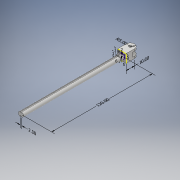
# Autodesk Inventor part: Tige
Saved by Autodesk Inventor 2018 (Build 220112000, 112)
## iProperties
Created: 2018-03-30
Part Number: Tige
Material: Générique
Document SubType Name: Modeling
Designer: Guadalix
Density: 1 g/cm^3
Appearance: Par défaut
Author: Guadalix
Autodesk Inventor part; units mm, degrees
ref_plane "YZ Plane" through (0, 0, 0) normal (1, 0, 0) x (0, 1, 0)
ref_plane "XZ Plane" through (0, 0, 0) normal (0, 1, 0) x (-1, 0, 0)
ref_plane "XY Plane" through (0, 0, 0) normal (0, 0, 1) x (1, 0, 0)
sketch "Esquisse1" plane through (0, 0, 0) normal (0, 0, 1) x (1, 0, 0)
  line L0 (-5, -5) -> (5, -5)
  line L1 (5, -5) -> (5, 5)
  line L2 (5, 5) -> (-5, 5)
  line L3 (-5, 5) -> (-5, -5)
  line L4 (-5, -5) -> (5, 5) construction
  line L5 (5, -5) -> (-5, 5) construction
  arc A0 (5, 5) -> (-5, 5) centre (0, 5) ccw
  point P0 (0, 0)
  dimension "d0" = 10
  dimension "d1" = 10
  constraints: 12 end point, 2 midpoint, 2 parallel, 2 point on circle, 1 centre point, 1 horizontal, 1 perpendicular, 1 tangent
  measures "d0" distance of L1.end L2.end
  measures "d1" distance of L0.end L1.end
extrude "Extrusion1" add sketch "Esquisse1" along normal blind 10
hole "Perçage1" at (0, 5, 10) direction (0, 0, -1) diameter 3 end through all
sketch "Esquisse3" plane through (0, 0, 0) normal (1, 0, 0) x (0, 1, 0)
  line L0 (15, 0) -> (15, 10)
  line L1 (3, 0) -> (3, 10)
  line L2 (15, 2.5) -> (3, 2.5)
  line L3 (3, 2.5) -> (3, 7.5)
  line L4 (3, 7.5) -> (15, 7.5)
  line L5 (15, 7.5) -> (15, 2.5)
  line L6 (15, 10) -> (3, 10)
  line L7 (15, 0) -> (3, 0)
  point P0 (0, 0)
  dimension "d23" = 12
  dimension "d29" = 5
  dimension "d30" = 2.5
  constraints: 16 end point, 2 parallel, 2 point on line, 1 horizontal, 1 perpendicular, 1 vertical, 2 other
  measures "d23" distance of L3.end L4.end
  measures "d29" distance between parallel lines of L2 L4
  measures "d30" distance of L4.end L0.end
extrude "Extrusion3" cut sketch "Esquisse3" along normal mid plane 100 contours L2 L1 L4 L0
sketch "Esquisse4" plane through (-5, -5, 0) normal (0, -1, 0) x (1, 0, 0)
  circle A0 centre (5, 5) radius 3
  line L0 (10, 0) -> (10, 10) projected
  line L1 (0, 10) -> (10, 10) projected
  line L2 (5, 8) -> (5, 2)
  line L3 (6, 7.8284) -> (6, 2.1716)
  line L4 (4, 7.8284) -> (4, 2.1716)
  line L5 (4, 6.8284) -> (6, 6.8284)
  line L6 (4, 3.1716) -> (6, 3.1716)
  point P0 (5, 0)
  point P1 (5, 6.8284)
  point P2 (4, 5)
  dimension "d24" = 6
  dimension "d25" = 5
  dimension "d26" = 5
  dimension "d37" = 2
  dimension "d38" = 1
  dimension "d39" = 1
  dimension "d40" = 1
  dimension "d41" = 1
  constraints: 10 end point, 6 point on circle, 5 point on line, 2 midpoint, 2 perpendicular, 2 vertical, 1 centre point, 1 coincident, 1 parallel
  measures "d24" diameter of A0
  measures "d25" distance from line of L0 A0.centre
  measures "d26" distance from line of L1 A0.centre
  measures "d37" distance of L5.start L5.end
  measures "d38" distance of L5.end point (5, 6.828)
  measures "d39" distance of point (4, 5) A0.centre
  measures "d40" distance of L4.start L5.start
  measures "d41" distance of L4.end L6.start
extrude "Extrusion4" add sketch "Esquisse4" along normal blind 120
extrude "Extrusion5" cut sketch "Esquisse4" along normal through all contours L3 L5 L2 A0 | A0 L2 L6 L3 | L2 L5 L4 A0 | A0 L4 L6 L2
